Autodesk Fusion 360 part; units mm, degrees
note: some values were not read from the file. Set by a fixed rule: which sketch regions a step uses.
(part 59 of 59)
  spline S76 degree 5 poles (26.8955, 23.4662) (26.8956, 23.4662) (26.8958, 23.4663) (26.8961, 23.4664) (26.8966, 23.4666) (26.8973, 23.4669) (26.8981, 23.4672) (26.899, 23.4676) (26.9, 23.4681) (26.9011, 23.4685) (26.9023, 23.4691) (26.9036, 23.4696) (26.905, 23.4702) (26.9065, 23.4709) (26.908, 23.4716) (26.9097, 23.4724) (26.9115, 23.4731) (26.9134, 23.474) (26.9153, 23.4749) (26.9173, 23.4758) (26.9195, 23.4768) (26.9217, 23.4778) (26.924, 23.4788) (26.9263, 23.4799) (26.9288, 23.4811) (26.9313, 23.4823) (26.9339, 23.4835) (26.9366, 23.4848) (26.9394, 23.4861) (26.9423, 23.4875) (26.9452, 23.4889) (26.9482, 23.4903) (26.9513, 23.4918) (26.9544, 23.4934) (26.9577, 23.4949) (26.961, 23.4966) (26.9643, 23.4982) (26.9678, 23.4999) (26.9713, 23.5017) (26.9748, 23.5035) (26.9785, 23.5053) (26.9822, 23.5072) (26.986, 23.5091) (26.9898, 23.5111) (26.9937, 23.5131) (26.9977, 23.5151) (27.0017, 23.5172) (27.0058, 23.5193) (27.01, 23.5215) (27.0142, 23.5237) (27.0185, 23.5259) (27.0228, 23.5282) (27.0272, 23.5306) (27.0317, 23.5329) (27.0362, 23.5353) (27.0408, 23.5378) (27.0454, 23.5403) (27.0501, 23.5428) (27.0549, 23.5454) (27.0597, 23.548) (27.0645, 23.5507) (27.0694, 23.5534) (27.0744, 23.5561) (27.0794, 23.5589) (27.0845, 23.5617) (27.0896, 23.5646) (27.0948, 23.5675) (27.1, 23.5704) (27.1053, 23.5734) (27.1106, 23.5764) (27.116, 23.5795) (27.1214, 23.5826) (27.1269, 23.5857) (27.1324, 23.5889) (27.138, 23.5921) (27.1436, 23.5954) (27.1493, 23.5987) (27.155, 23.602) (27.1608, 23.6054) (27.1666, 23.6088) (27.1725, 23.6123) (27.1784, 23.6158) (27.1843, 23.6193) (27.1903, 23.6229) (27.1963, 23.6265) (27.2024, 23.6301) (27.2085, 23.6338) (27.2147, 23.6376) (27.2209, 23.6413) (27.2271, 23.6451) (27.2334, 23.649) (27.2397, 23.6529) (27.2461, 23.6568) (27.2525, 23.6608) (27.259, 23.6648) (27.2654, 23.6688) (27.272, 23.6729) (27.2785, 23.677) (27.2851, 23.6812) (27.2918, 23.6854) (27.2985, 23.6896) (27.3052, 23.6939) (27.3119, 23.6982) (27.3187, 23.7025) (27.3256, 23.7069) (27.3324, 23.7113) (27.3393, 23.7158) (27.3463, 23.7203) (27.3533, 23.7248) (27.3603, 23.7294) (27.3673, 23.734) (27.3744, 23.7387) (27.3815, 23.7434) (27.3887, 23.7481) (27.3958, 23.7529) (27.4031, 23.7577) (27.4103, 23.7625) (27.4176, 23.7674) (27.4249, 23.7723) (27.4323, 23.7773) (27.4396, 23.7823) (27.447, 23.7873) (27.4545, 23.7924) (27.462, 23.7975) (27.4695, 23.8026) (27.477, 23.8078) (27.4846, 23.813) (27.4922, 23.8183) (27.4998, 23.8235) (27.5074, 23.8289) (27.5151, 23.8342) (27.5228, 23.8396) (27.5306, 23.8451) (27.5384, 23.8506) (27.5462, 23.8561) (27.554, 23.8616) (27.5618, 23.8672) (27.5697, 23.8728) (27.5776, 23.8785) (27.5856, 23.8842) (27.5936, 23.8899) (27.6015, 23.8957) (27.6096, 23.9015) (27.6176, 23.9074) (27.6257, 23.9132) (27.6338, 23.9192) (27.6419, 23.9251) (27.6501, 23.9311) (27.6582, 23.9371) (27.6665, 23.9432) (27.6747, 23.9493) (27.6829, 23.9554) (27.6912, 23.9616) (27.6995, 23.9678) (27.7078, 23.9741) (27.7162, 23.9803) (27.7246, 23.9867) (27.733, 23.993) (27.7414, 23.9994) (27.7498, 24.0058) (27.7583, 24.0123) (27.7668, 24.0188) (27.7753, 24.0253) (27.7838, 24.0319) (27.7924, 24.0385) (27.801, 24.0452) (27.8096, 24.0518) (27.8182, 24.0585) (27.8268, 24.0653) (27.8355, 24.0721) (27.8442, 24.0789) (27.8529, 24.0858) (27.8616, 24.0927) (27.8704, 24.0996) (27.8791, 24.1065) (27.8879, 24.1135) (27.8967, 24.1206) (27.9055, 24.1276) (27.9144, 24.1348) (27.9233, 24.1419) (27.9322, 24.1491) (27.9411, 24.1563) (27.95, 24.1635) (27.9589, 24.1708) (27.9679, 24.1781) (27.9769, 24.1855) (27.9859, 24.1929) (27.9949, 24.2003) (28.0039, 24.2078) (28.013, 24.2153) (28.0221, 24.2228) (28.0312, 24.2303) (28.0403, 24.2379) (28.0494, 24.2456) (28.0585, 24.2532) (28.0677, 24.2609) (28.0769, 24.2687) (28.0861, 24.2765) (28.0953, 24.2843) (28.1045, 24.2921) (28.1137, 24.3) (28.123, 24.3079) (28.1323, 24.3158) (28.1416, 24.3238) (28.1509, 24.3318) (28.1602, 24.3399) (28.1695, 24.348) (28.1789, 24.3561) (28.1882, 24.3643) (28.1976, 24.3724) (28.207, 24.3807) (28.2164, 24.3889) (28.2259, 24.3972) (28.2353, 24.4055) (28.2447, 24.4139) (28.2542, 24.4223) (28.2637, 24.4307) (28.2732, 24.4392) (28.2827, 24.4477) (28.2922, 24.4562) (28.3018, 24.4648) (28.3113, 24.4734) (28.3209, 24.482) (28.3305, 24.4907) (28.34, 24.4994) (28.3496, 24.5081) (28.3593, 24.5169) (28.3689, 24.5257) (28.3785, 24.5345) (28.3882, 24.5434) (28.3978, 24.5523) (28.4075, 24.5613) (28.4172, 24.5702) (28.4269, 24.5792) (28.4366, 24.5883) (28.4464, 24.5973) (28.4561, 24.6065) (28.4658, 24.6156) (28.4756, 24.6248) (28.4854, 24.634) (28.4951, 24.6432) (28.503, 24.6506) (28.5089, 24.6562) (28.5128, 24.66) (28.5147, 24.6618) knots 0 0 0 0 0 0 0.00416667 0.00833333 0.0125 0.01666667 0.02083333 0.025 0.02916667 0.03333333 0.0375 0.04166667 0.04583333 0.05 0.05416667 0.05833333 0.0625 0.06666667 0.07083333 0.075 0.07916667 0.08333333 0.0875 0.09166667 0.09583333 0.1 0.10416667 0.10833333 0.1125 0.11666667 0.12083333 0.125 0.12916667 0.13333333 0.1375 0.14166667 0.14583333 0.15 0.15416667 0.15833333 0.1625 0.16666667 0.17083333 0.175 0.17916667 0.18333333 0.1875 0.19166667 0.19583333 0.2 0.20416667 0.20833333 0.2125 0.21666667 0.22083333 0.225 0.22916667 0.23333333 0.2375 0.24166667 0.24583333 0.25 0.25416667 0.25833333 0.2625 0.26666667 0.27083333 0.275 0.27916667 0.28333333 0.2875 0.29166667 0.29583333 0.3 0.30416667 0.30833333 0.3125 0.31666667 0.32083333 0.325 0.32916667 0.33333333 0.3375 0.34166667 0.34583333 0.35 0.35416667 0.35833333 0.3625 0.36666667 0.37083333 0.375 0.37916667 0.38333333 0.3875 0.39166667 0.39583333 0.4 0.40416667 0.40833333 0.4125 0.41666667 0.42083333 0.425 0.42916667 0.43333333 0.4375 0.44166667 0.44583333 0.45 0.45416667 0.45833333 0.4625 0.46666667 0.47083333 0.475 0.47916667 0.48333333 0.4875 0.49166667 0.49583333 0.5 0.50416667 0.50833333 0.5125 0.51666667 0.52083333 0.525 0.52916667 0.53333333 0.5375 0.54166667 0.54583333 0.55 0.55416667 0.55833333 0.5625 0.56666667 0.57083333 0.575 0.57916667 0.58333333 0.5875 0.59166667 0.59583333 0.6 0.60416667 0.60833333 0.6125 0.61666667 0.62083333 0.625 0.62916667 0.63333333 0.6375 0.64166667 0.64583333 0.65 0.65416667 0.65833333 0.6625 0.66666667 0.67083333 0.675 0.67916667 0.68333333 0.6875 0.69166667 0.69583333 0.7 0.70416667 0.70833333 0.7125 0.71666667 0.72083333 0.725 0.72916667 0.73333333 0.7375 0.74166667 0.74583333 0.75 0.75416667 0.75833333 0.7625 0.76666667 0.77083333 0.775 0.77916667 0.78333333 0.7875 0.79166667 0.79583333 0.8 0.80416667 0.80833333 0.8125 0.81666667 0.82083333 0.825 0.82916667 0.83333333 0.8375 0.84166667 0.84583333 0.85 0.85416667 0.85833333 0.8625 0.86666667 0.87083333 0.875 0.87916667 0.88333333 0.8875 0.89166667 0.89583333 0.9 0.90416667 0.90833333 0.9125 0.91666667 0.92083333 0.925 0.92916667 0.93333333 0.9375 0.94166667 0.94583333 0.95 0.95416667 0.95833333 0.9625 0.96666667 0.97083333 0.975 0.97916667 0.98333333 0.9875 0.99166667 0.99583333 1 1 1 1 1 1
  arc A77 (28.5147, 24.6618) -> (28.1181, 25.5527) centre (0, 12.5) ccw
  spline S77 degree 5 poles (28.1181, 25.5527) (28.1154, 25.5525) (28.11, 25.5521) (28.1019, 25.5515) (28.0911, 25.5506) (28.0777, 25.5495) (28.0644, 25.5484) (28.051, 25.5473) (28.0377, 25.5462) (28.0244, 25.5451) (28.0112, 25.5439) (27.9979, 25.5427) (27.9848, 25.5415) (27.9716, 25.5404) (27.9585, 25.5391) (27.9454, 25.5379) (27.9323, 25.5367) (27.9193, 25.5354) (27.9063, 25.5342) (27.8934, 25.5329) (27.8805, 25.5316) (27.8676, 25.5303) (27.8547, 25.529) (27.8419, 25.5276) (27.8291, 25.5263) (27.8164, 25.5249) (27.8037, 25.5236) (27.791, 25.5222) (27.7784, 25.5208) (27.7658, 25.5194) (27.7532, 25.518) (27.7406, 25.5165) (27.7281, 25.5151) (27.7157, 25.5136) (27.7032, 25.5122) (27.6908, 25.5107) (27.6785, 25.5092) (27.6661, 25.5077) (27.6539, 25.5062) (27.6416, 25.5047) (27.6294, 25.5031) (27.6172, 25.5016) (27.605, 25.5) (27.5929, 25.4984) (27.5809, 25.4968) (27.5688, 25.4952) (27.5568, 25.4936) (27.5449, 25.492) (27.5329, 25.4904) (27.521, 25.4887) (27.5092, 25.4871) (27.4974, 25.4854) (27.4856, 25.4838) (27.4738, 25.4821) (27.4621, 25.4804) (27.4505, 25.4787) (27.4388, 25.477) (27.4273, 25.4752) (27.4157, 25.4735) (27.4042, 25.4718) (27.3927, 25.47) (27.3813, 25.4682) (27.3699, 25.4665) (27.3585, 25.4647) (27.3472, 25.4629) (27.3359, 25.4611) (27.3247, 25.4593) (27.3135, 25.4574) (27.3023, 25.4556) (27.2912, 25.4538) (27.2801, 25.4519) (27.2691, 25.4501) (27.2581, 25.4482) (27.2471, 25.4463) (27.2362, 25.4445) (27.2253, 25.4426) (27.2145, 25.4407) (27.2037, 25.4388) (27.1929, 25.4368) (27.1822, 25.4349) (27.1715, 25.433) (27.1609, 25.4311) (27.1503, 25.4291) (27.1397, 25.4272) (27.1292, 25.4252) (27.1188, 25.4232) (27.1083, 25.4213) (27.0979, 25.4193) (27.0876, 25.4173) (27.0773, 25.4153) (27.0671, 25.4133) (27.0568, 25.4113) (27.0467, 25.4093) (27.0365, 25.4072) (27.0265, 25.4052) (27.0164, 25.4032) (27.0064, 25.4011) (26.9965, 25.3991) (26.9866, 25.3971) (26.9767, 25.395) (26.9669, 25.3929) (26.9571, 25.3909) (26.9474, 25.3888) (26.9377, 25.3867) (26.9281, 25.3847) (26.9185, 25.3826) (26.9089, 25.3805) (26.8994, 25.3784) (26.89, 25.3763) (26.8806, 25.3742) (26.8712, 25.3721) (26.8619, 25.37) (26.8526, 25.3679) (26.8434, 25.3658) (26.8342, 25.3636) (26.8251, 25.3615) (26.816, 25.3594) (26.8069, 25.3573) (26.798, 25.3551) (26.789, 25.353) (26.7801, 25.3509) (26.7713, 25.3487) (26.7625, 25.3466) (26.7537, 25.3445) (26.7451, 25.3423) (26.7364, 25.3402) (26.7278, 25.338) (26.7193, 25.3359) (26.7108, 25.3337) (26.7023, 25.3316) (26.6939, 25.3294) (26.6856, 25.3273) (26.6773, 25.3251) (26.669, 25.323) (26.6608, 25.3208) (26.6527, 25.3187) (26.6446, 25.3166) (26.6365, 25.3144) (26.6286, 25.3123) (26.6206, 25.3101) (26.6127, 25.308) (26.6049, 25.3058) (26.5971, 25.3037) (26.5894, 25.3016) (26.5817, 25.2994) (26.5741, 25.2973) (26.5665, 25.2952) (26.559, 25.293) (26.5516, 25.2909) (26.5442, 25.2888) (26.5368, 25.2867) (26.5296, 25.2845) (26.5223, 25.2824) (26.5151, 25.2803) (26.508, 25.2782) (26.5009, 25.2761) (26.4939, 25.274) (26.487, 25.272) (26.4801, 25.2699) (26.4733, 25.2678) (26.4665, 25.2657) (26.4598, 25.2637) (26.4531, 25.2616) (26.4465, 25.2596) (26.4399, 25.2575) (26.4335, 25.2555) (26.427, 25.2534) (26.4207, 25.2514) (26.4144, 25.2494) (26.4081, 25.2474) (26.4019, 25.2454) (26.3958, 25.2434) (26.3897, 25.2414) (26.3837, 25.2395) (26.3778, 25.2375) (26.3719, 25.2356) (26.3661, 25.2336) (26.3604, 25.2317) (26.3547, 25.2298) (26.3491, 25.2279) (26.3435, 25.226) (26.338, 25.2241) (26.3326, 25.2222) (26.3273, 25.2204) (26.322, 25.2185) (26.3167, 25.2167) (26.3116, 25.2149) (26.3065, 25.2131) (26.3015, 25.2113) (26.2965, 25.2095) (26.2916, 25.2077) (26.2868, 25.206) (26.282, 25.2043) (26.2774, 25.2026) (26.2728, 25.2009) (26.2682, 25.1992) (26.2638, 25.1975) (26.2594, 25.1959) (26.255, 25.1943) (26.2508, 25.1927) (26.2466, 25.1911) (26.2425, 25.1895) (26.2385, 25.188) (26.2345, 25.1864) (26.2307, 25.1849) (26.2269, 25.1834) (26.2231, 25.182) (26.2195, 25.1806) (26.2159, 25.1791) (26.2124, 25.1778) (26.209, 25.1764) (26.2057, 25.175) (26.2024, 25.1737) (26.1993, 25.1724) (26.1962, 25.1712) (26.1932, 25.1699) (26.1903, 25.1687) (26.1874, 25.1676) (26.1847, 25.1664) (26.182, 25.1653) (26.1794, 25.1642) (26.1769, 25.1631) (26.1745, 25.1621) (26.1722, 25.1611) (26.17, 25.1602) (26.1678, 25.1592) (26.1658, 25.1583) (26.1638, 25.1575) (26.1619, 25.1567) (26.1602, 25.1559) (26.1585, 25.1551) (26.1569, 25.1544) (26.1554, 25.1538) (26.154, 25.1531) (26.1527, 25.1526) (26.1515, 25.152) (26.1504, 25.1515) (26.1495, 25.151) (26.1486, 25.1506) (26.1478, 25.1503) (26.1471, 25.15) (26.1467, 25.1497) (26.1464, 25.1496) (26.1462, 25.1495) (26.1461, 25.1495) knots -1 -1 -1 -1 -1 -1 -0.99583333 -0.99166667 -0.9875 -0.98333333 -0.97916667 -0.975 -0.97083333 -0.96666667 -0.9625 -0.95833333 -0.95416667 -0.95 -0.94583333 -0.94166667 -0.9375 -0.93333333 -0.92916667 -0.925 -0.92083333 -0.91666667 -0.9125 -0.90833333 -0.90416667 -0.9 -0.89583333 -0.89166667 -0.8875 -0.88333333 -0.87916667 -0.875 -0.87083333 -0.86666667 -0.8625 -0.85833333 -0.85416667 -0.85 -0.84583333 -0.84166667 -0.8375 -0.83333333 -0.82916667 -0.825 -0.82083333 -0.81666667 -0.8125 -0.80833333 -0.80416667 -0.8 -0.79583333 -0.79166667 -0.7875 -0.78333333 -0.77916667 -0.775 -0.77083333 -0.76666667 -0.7625 -0.75833333 -0.75416667 -0.75 -0.74583333 -0.74166667 -0.7375 -0.73333333 -0.72916667 -0.725 -0.72083333 -0.71666667 -0.7125 -0.70833333 -0.70416667 -0.7 -0.69583333 -0.69166667 -0.6875 -0.68333333 -0.67916667 -0.675 -0.67083333 -0.66666667 -0.6625 -0.65833333 -0.65416667 -0.65 -0.64583333 -0.64166667 -0.6375 -0.63333333 -0.62916667 -0.625 -0.62083333 -0.61666667 -0.6125 -0.60833333 -0.60416667 -0.6 -0.59583333 -0.59166667 -0.5875 -0.58333333 -0.57916667 -0.575 -0.57083333 -0.56666667 -0.5625 -0.55833333 -0.55416667 -0.55 -0.54583333 -0.54166667 -0.5375 -0.53333333 -0.52916667 -0.525 -0.52083333 -0.51666667 -0.5125 -0.50833333 -0.50416667 -0.5 -0.49583333 -0.49166667 -0.4875 -0.48333333 -0.47916667 -0.475 -0.47083333 -0.46666667 -0.4625 -0.45833333 -0.45416667 -0.45 -0.44583333 -0.44166667 -0.4375 -0.43333333 -0.42916667 -0.425 -0.42083333 -0.41666667 -0.4125 -0.40833333 -0.40416667 -0.4 -0.39583333 -0.39166667 -0.3875 -0.38333333 -0.37916667 -0.375 -0.37083333 -0.36666667 -0.3625 -0.35833333 -0.35416667 -0.35 -0.34583333 -0.34166667 -0.3375 -0.33333333 -0.32916667 -0.325 -0.32083333 -0.31666667 -0.3125 -0.30833333 -0.30416667 -0.3 -0.29583333 -0.29166667 -0.2875 -0.28333333 -0.27916667 -0.275 -0.27083333 -0.26666667 -0.2625 -0.25833333 -0.25416667 -0.25 -0.24583333 -0.24166667 -0.2375 -0.23333333 -0.22916667 -0.225 -0.22083333 -0.21666667 -0.2125 -0.20833333 -0.20416667 -0.2 -0.19583333 -0.19166667 -0.1875 -0.18333333 -0.17916667 -0.175 -0.17083333 -0.16666667 -0.1625 -0.15833333 -0.15416667 -0.15 -0.14583333 -0.14166667 -0.1375 -0.13333333 -0.12916667 -0.125 -0.12083333 -0.11666667 -0.1125 -0.10833333 -0.10416667 -0.1 -0.09583333 -0.09166667 -0.0875 -0.08333333 -0.07916667 -0.075 -0.07083333 -0.06666667 -0.0625 -0.05833333 -0.05416667 -0.05 -0.04583333 -0.04166667 -0.0375 -0.03333333 -0.02916667 -0.025 -0.02083333 -0.01666667 -0.0125 -0.00833333 -0.00416667 0 0 0 0 0 0
  line L155 (26.1461, 25.1495) -> (26.1453, 25.1491)
  line L156 (26.1453, 25.1491) -> (25.8803, 25.0209)
  line L157 (25.8803, 25.0209) -> (19, 25)
  line L158 (19, 25) -> (19, 45)
  line L159 (19, 45) -> (11, 45)
  line L160 (11, 45) -> (11, 25)
  line L161 (11, 25) -> (-11, 25)
  line L162 (-11, 25) -> (-11, 45)
  line L163 (-11, 45) -> (-19, 45)
  line L164 (-19, 45) -> (-19, 25)
  circle A78 centre (0, 12.5) radius 8
  circle A79 centre (0, 12.5) radius 10
  line L165 (0, 12.5) -> (-10, 12.5)
  line L166 (0, 12.5) -> (0, 2.5)
  line L167 (0, 12.5) -> (0, 22.5)
  circle A80 centre (-10, 12.5) radius 1.25
  line L168 (0, 12.5) -> (10, 12.5)
  circle A81 centre (10, 12.5) radius 1.25
  circle A82 centre (0, 2.5) radius 1.25
  circle A83 centre (0, 22.5) radius 1.25
  dimension "d124" = 16
  dimension "d125" = 20
  dimension "d126" = 2.5
  dimension "d128" = 2.5
  dimension "d129" = 2.5
  dimension "d130" = 2.5
  constraint concentric A0 A78
  constraint concentric A78 A79
  constraint coincident A0.centre A1.centre
  constraint coincident A79 L165.end
  constraint horizontal L165
  constraint coincident A79 L166.end
  constraint perpendicular L165 L166
  constraint coincident A79 L167.end
  constraint perpendicular L165 L167
  constraint coincident L165.end A80.centre
  constraint coincident A79 L168.end
  constraint perpendicular L167 L168
  constraint coincident L168.end A81.centre
  constraint coincident L166.end A82.centre
  constraint coincident L167.end A83.centre
  measures "d124" diameter of A78
  measures "d125" diameter of A79
  measures "d126" diameter of A80
  measures "d128" diameter of A81
  measures "d129" diameter of A82
  measures "d130" diameter of A83
extrude "押し出し20" cut sketch "スケッチ25" against normal blind 8 contours A79 L168 A81 | A79 L168 A81 | A79 L167 A83 | A79 L167 A83 | A79 L166 A82 | A79 L166 A82 | A79 A81 | A79 L165 A80 | A79 L165 A80 | A79 A83 | A79 A82 | A79 A80
